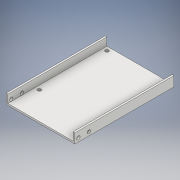
# Autodesk Inventor part: learnbotAgarreOdroid
Saved by Autodesk Inventor 2017 (Build 210142000, 142)
## iProperties
Part Number: learnbotAgarreOdroid
Material: Genérico
Document SubType Name: Modeling
Designer: rober
Density: 1 g/cm^3
Appearance: Valor por defecto
Author: rober
Autodesk Inventor part; units mm, degrees
ref_plane "YZ Plane" through (0, 0, 0) normal (1, 0, 0) x (0, 1, 0)
ref_plane "XZ Plane" through (0, 0, 0) normal (0, 1, 0) x (-1, 0, 0)
ref_plane "XY Plane" through (0, 0, 0) normal (0, 0, 1) x (1, 0, 0)
sketch "Boceto1" plane through (0, 0, 0) normal (0, 0, 1) x (1, 0, 0)
  line L0 (0.15, 0) -> (0, 0)
  line L1 (0, 0) -> (0, 8.5)
  line L2 (0, 8.5) -> (0.15, 8.5)
  line L3 (0.15, 8.5) -> (0.15, 0)
  line L4 (0.15, 0) -> (5.9, 0)
  line L5 (5.9, 0) -> (5.9, 8.5)
  line L6 (5.9, 8.5) -> (5.75, 8.5)
  line L7 (5.75, 8.5) -> (5.6932, 0)
  line L8 (5.75, 8.5) -> (0.15, 8.5)
  circle A0 centre (0.5, 2.35) radius 0.15
  circle A1 centre (5.4, 2.35) radius 0.15
  circle A2 centre (0.5, 8.15) radius 0.15
  circle A3 centre (5.4, 8.15) radius 0.15
  constraints: 18 end point, 4 centre point, 1 point on line
extrude "Extrusión1" add sketch "Boceto1" along normal blind 0.15
sketch "Boceto2" plane through (5.9, 0, 0) normal (1, 0, 0) x (0, 0, -1)
  line L0 (0, 0) -> (0, 8.5)
  line L1 (0, 8.5) -> (-0.8328, 8.5)
  line L2 (-0.8328, 8.5) -> (-0.8328, 0)
  line L3 (-0.8328, 0) -> (0, 0)
  circle A0 centre (-0.3164, 0.3) radius 0.15
  circle A1 centre (-0.3164, 1.2) radius 0.15
  line L4 (0, 8.5) -> (-0.15, 8.5)
  line L5 (-0.15, 8.5) -> (-0.15, 0)
  constraints: 12 end point, 2 centre point, 2 point on line
extrude "Extrusión2" add sketch "Boceto2" against normal blind 0.15 contours L3 L2 L1 L5
sketch "Boceto3" plane through (0, 0, 0) normal (-1, 0, 0) x (0, 0, 1)
  line L0 (0, 0) -> (0, 8.5)
  line L1 (0, 8.5) -> (0.8328, 8.5)
  line L2 (0.8328, 8.5) -> (0.8328, 0)
  line L3 (0.8328, 0) -> (0, 0)
  circle A0 centre (0.3164, 0.3) radius 0.15
  circle A1 centre (0.3164, 1.2) radius 0.15
  line L4 (0, 8.5) -> (0.15, 8.5)
  line L5 (0.15, 8.5) -> (0.15, 0)
  constraints: 12 end point, 2 centre point, 2 point on line
extrude "Extrusión3" add sketch "Boceto3" against normal blind 0.15 contours L5 L1 L2 L3
